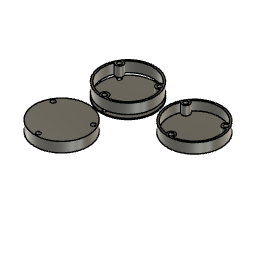
Basic Elements Generator v3 (Autodesk Fusion 360 design; units mm, degrees)
Autodesk Fusion 360 part; units mm, degrees
sketch "Schizzo1" plane through (0, 0, 0) normal (0, 0, 1) x (1, 0, 0)
  circle A0 centre (-60.6218, 35) radius 6.1
  line L0 (-60.6218, 35) -> (0, -70) construction
  line L1 (0, -70) -> (60.6218, 35) construction
  circle A1 centre (0, -70) radius 6.1
  circle A2 centre (60.6218, 35) radius 6.3
  circle A3 centre (-60.6218, 35) radius 6.3
  circle A4 centre (0, 0) radius 80
  line L2 (60.6218, 35) -> (-60.6218, 35) construction
  circle A5 centre (0, 0) radius 70 construction
  circle A6 centre (60.6218, 35) radius 6.1
  circle A7 centre (0, -70) radius 6.3
  line L3 (0, 0) -> (0, -70) construction
  line L4 (-100, -136.5722) -> (-100, 127.6789) construction
  line L5 (-139.3782, 35) -> (-200, -70) construction
  circle A8 centre (-260.6218, 35) radius 6.3
  line L6 (-200, 0) -> (-200, -70) construction
  line L7 (-200, -70) -> (-260.6218, 35) construction
  line L8 (-260.6218, 35) -> (-139.3782, 35) construction
  circle A9 centre (-139.3782, 35) radius 6.3
  circle A10 centre (-200, -70) radius 6.3
  circle A11 centre (-200, -70) radius 6.1
  circle A12 centre (-200, 0) radius 80
  circle A13 centre (-139.3782, 35) radius 6.1
  circle A14 centre (-200, 0) radius 70 construction
  circle A15 centre (-260.6218, 35) radius 6.1
  point P0 (-200, 0)
  point P1 (-200, 0)
  dimension "d1" = 140
  dimension "d2" = 10
  dimension "d3" = 0.2
  dimension "d4" = 12.2
  dimension "d17" = 100
  constraint coincident A4.centre A5.centre
  constraint coincident L0.end A5
  constraint vertical L3
  constraint coincident L0.end L1.start
  constraint coincident L1.end A5
  constraint coincident A0.centre A5
  constraint horizontal L2
  constraint equal L1 L2
  constraint coincident L1.end A2.centre
  constraint coincident A0.centre L0.start
  constraint equal A3 A7
  constraint equal A2 A7
  constraint concentric A0 A3
  constraint concentric A1 A7
  constraint concentric A2 A6
  constraint equal A1 A6
  constraint equal A0 A1
  constraint parallel L3 L4
  constraint symmetric A4.centre L4 P1
  constraint symmetric L0.end L4 L5.end
  constraint symmetric A0.centre L4 L5.start
  constraint symmetric L1.end L4 A8.centre
  constraint symmetric A0 L4 A13
  constraint symmetric A1 L4 A11
  constraint symmetric A2 L4 A8
  constraint symmetric A3 L4 A9
  constraint symmetric A4 L4 A12
  constraint symmetric A5 L4 A14
  constraint symmetric A6 L4 A15
  constraint symmetric A7 L4 A10
  measures "d1" diameter of A5
  measures "d2" distance of A4 A5
  measures "d3" distance of A1 A7
  measures "d4" diameter of A1
  measures "d17" distance of A4.centre L4
extrude "Estrusione2" add sketch "Schizzo1" along normal blind 27 contours A4 makes body 1
shell "Svuotamento1" thickness 5 removed faces 2 at (-0.1569, -0.2718, 27) at (-0.1569, -0.2718, 0) on bodies 1
extrude "Estrusione1" add sketch "Schizzo1" against normal blind 3 contours A4 bodies 1
extrude "Estrusione4" add sketch "Schizzo1" along normal blind 30 separate body contours A12 makes body 2
copy_body "CopiaIncollaCorpi1" bodies 2 makes body 3
move_body "Sposta1" bodies 3 to x (1, 0, 0) y (0, 1, 0) z (0, 0, 1) at (0, -200, 0)
shell "Svuotamento2" thickness 5 removed faces 2 at (-200.1569, 0.2718, 30) at (-200.1569, 0.2718, 0) on bodies 2
extrude "Estrusione5" add sketch "Schizzo1" against normal blind 3 from surface at -10 separate body contours A12 makes body 4
equation "Floor_Thickness = 3 mm"
equation "Wall_Thickness = 5 mm"
equation "Height = 30 mm" comment "Will include Floor_Thickness in the \"complete\" body"
equation "d8 = -Floor_Thickness"
equation "d10 = Height - Floor_Thickness"
equation "d12 = Wall_Thickness"
equation "Roof_Thickness = 0 mm"
equation "d18 = Height"
equation "d20 = Wall_Thickness"
equation "d22 = -Floor_Thickness"
named bodies: "Complete", "Wall only", "Floor only", "Solid"
